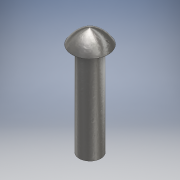
# Autodesk Inventor part: m3_bolt
Saved by Autodesk Inventor 2017 (Build 210142000, 142)
## iProperties
Created: 2018-04-08
Part Number: m3_bolt
Material: Steel, Galvanized
Document SubType Name: Modeling
Designer: Roland
Density: 7.85 g/cm^3
Appearance: Galvanized
Author: Roland
Autodesk Inventor part; units mm, degrees
ref_plane "YZ Plane" through (0, 0, 0) normal (1, 0, 0) x (0, 1, 0)
ref_plane "XZ Plane" through (0, 0, 0) normal (0, 1, 0) x (-1, 0, 0)
ref_plane "XY Plane" through (0, 0, 0) normal (0, 0, 1) x (1, 0, 0)
sketch "Sketch1" plane through (0, 0, 0) normal (0, 0, 1) x (1, 0, 0)
  circle A0 centre (0, 0) radius 1.5
  dimension "d0" = 3
  constraints: 1 centre point, 1 coincident
  measures "d0" diameter of A0
extrude "Extrusion1" add sketch "Sketch1" along normal blind 13
sketch "Sketch2" plane through (0, 0, 0) normal (1, 0, 0) x (0, 1, 0)
  line L0 (1.5, 13) -> (-1.5, 13) projected
  line L1 (0, 13) -> (0, 15)
  line L2 (0, 13) -> (2.5, 13)
  arc A0 (2.5, 13) -> (0, 15) centre (-1.3597, 10.7379) ccw
  point P0 (0, 0)
  dimension "d3" = 2.5
  constraints: 4 end point, 2 point on circle, 1 centre point, 1 midpoint, 1 point on line
  measures "d3" distance of L1.start L2.end
revolve "Revolution1" add sketch "Sketch2" angle 360 about axis through (0, 0, 13) along (0, 0, 1)
body "Solid1"
